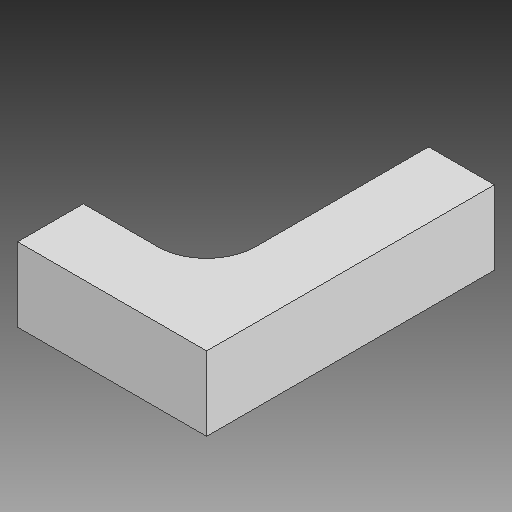
# Autodesk Inventor part: angle
Saved by Autodesk Inventor 2026 (Build 300175000, 175)
## iProperties
Created: 2025-10-18
Part Number: angle
Material: Типовые
Document SubType Name: Modeling
Designer: Admin
Density: 1 g/cm^3
Appearance: По умолчанию
Author: Admin
Autodesk Inventor part; units mm, degrees
ref_plane "YZ Plane" through (0, 0, 0) normal (1, 0, 0) x (0, 1, 0)
ref_plane "XZ Plane" through (0, 0, 0) normal (0, 1, 0) x (-1, 0, 0)
ref_plane "XY Plane" through (0, 0, 0) normal (0, 0, 1) x (1, 0, 0)
sketch "Эскиз1" plane through (0, 0, 0) normal (0, 1, 0) x (-1, 0, 0)
  line L0 (-4, 17.5) -> (4, 17.5)
  line L1 (4, 3.5) -> (4, -17.5)
  line L2 (4, -17.5) -> (-4, -17.5)
  line L3 (-4, -17.5) -> (-4, 17.5)
  line L4 (-4, 17.5) -> (4, -17.5) construction
  line L5 (4, 17.5) -> (-4, -17.5) construction
  line L6 (4, 17.5) -> (19, 17.5)
  line L7 (19, 17.5) -> (19, 9.5)
  line L8 (19, 9.5) -> (10, 9.5)
  arc A0 (10, 9.5) -> (4, 3.5) centre (10, 3.5) ccw
  point P0 (0, 0)
  point P1 (4, 9.5)
  dimension "d0" = 8
  dimension "d2" = 15
  dimension "d3" = 8
  dimension "d4" = 35
  dimension "d5" = 6
  constraints: 18 end point, 3 parallel, 2 horizontal, 2 midpoint, 2 perpendicular, 2 point on circle, 2 point on line, 2 tangent, 1 centre point
  measures "d0" distance of L1.end L2.end
  measures "d2" distance of point (4, 9.5) L7.end
  measures "d3" distance of L6.end L7.end
  measures "d4" distance of L2.end L0.start
  measures "d5" radius of A0
extrude "Выдавливание1" add sketch "Эскиз1" along normal blind 9
